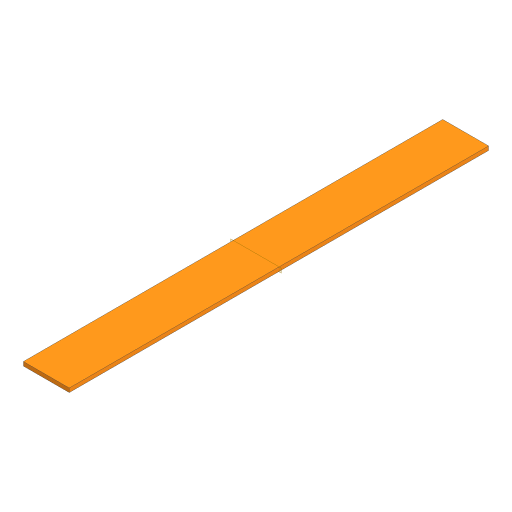
# Autodesk Inventor part: Фанера крыла
Saved by Autodesk Inventor 2023.2 (Build 272271030, 271C)
## iProperties
Created: 2025-02-01
Part Number: Фанера крыла
Material: Типовые
Document SubType Name: Modeling
Designer: Коноваленко
Density: 1 g/cm^3
Appearance: По умолчанию
Author: Коноваленко
Autodesk Inventor part; units mm, degrees
ref_plane "YZ Plane" through (0, 0, 0) normal (1, 0, 0) x (0, 1, 0)
ref_plane "XZ Plane" through (0, 0, 0) normal (0, 1, 0) x (-1, 0, 0)
sketch "Эскиз1" plane through (0, 0, 0) normal (0, 1, 0) x (-1, 0, 0)
  line L0 (17.5, -160) -> (-17.5, -160)
  line L1 (-17.5, -160) -> (-17.5, 160)
  line L2 (-17.5, 160) -> (17.5, 160)
  line L3 (17.5, 160) -> (17.5, -160)
  line L4 (0, -224) -> (0, 224) projected
  line L5 (-24.5, 0) -> (24.5, 0) projected
  point P0 (0, 0)
  point P1 (0, -160)
  point P2 (17.5, 0)
  dimension "d0" = 35
  dimension "d1" = 320
  constraints: 8 end point, 2 midpoint, 2 parallel, 2 point on line, 1 horizontal, 1 perpendicular
  measures "d0" distance between parallel lines of L1 L3
  measures "d1" distance between parallel lines of L2 L0
extrude "Выдавливание1" add sketch "Эскиз1" along normal mid plane 3
